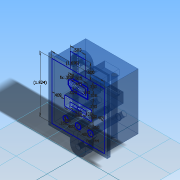
# Autodesk Inventor part: PanelMountNew
Saved by Autodesk Inventor 2014 SP2 (Build 180246200, 246)
## iProperties
Created: 2014-06-07
Part Number: PanelMountNew
Material: Generic
Document SubType Name: Modeling
Designer: dliu
Density: 1 g/cm^3
Appearance: Default
Author: dliu
Autodesk Inventor part; units mm, degrees
ref_plane "YZ Plane" through (0, 0, 0) normal (1, 0, 0) x (0, 1, 0)
ref_plane "XZ Plane" through (0, 0, 0) normal (0, 1, 0) x (-1, 0, 0)
sketch "Sketch1" plane through (0, 0, 0) normal (0, 0, 1) x (1, 0, 0)
  line L0 (7.6835, 18.4404) -> (7.6835, 10.414)
  line L1 (-7.6835, 15.9004) -> (-5.1435, 18.4404)
  line L2 (-7.6835, 12.954) -> (-5.1435, 10.414)
  line L3 (-7.6835, 12.954) -> (-7.6835, 15.9004)
  line L4 (-5.1435, 18.4404) -> (7.6835, 18.4404)
  line L5 (7.6835, 10.414) -> (-5.1435, 10.414)
  line L6 (-5.9055, 12.0142) -> (5.9055, 12.0142)
  line L7 (5.9055, 12.0142) -> (5.9055, 16.8402)
  line L8 (5.9055, 16.8402) -> (-5.9055, 16.8402)
  line L9 (-5.9055, 16.8402) -> (-5.9055, 12.0142)
  line L10 (-11.176, 4.064) -> (11.176, 4.064)
  line L11 (11.176, 4.064) -> (11.176, -4.064)
  line L12 (11.176, -4.064) -> (-11.176, -4.064)
  line L13 (-11.176, -4.064) -> (-11.176, 4.064)
  line L14 (-11.176, 4.064) -> (11.176, -4.064) construction
  line L15 (11.176, 4.064) -> (-11.176, -4.064) construction
  line L16 (-6.604, 1.27) -> (6.604, 1.27)
  line L17 (6.604, 1.27) -> (6.604, -1.27)
  line L18 (6.604, -1.27) -> (-6.604, -1.27)
  line L19 (-6.604, -1.27) -> (-6.604, 1.27)
  line L20 (-6.604, 1.27) -> (6.604, -1.27) construction
  line L21 (6.604, 1.27) -> (-6.604, -1.27) construction
  circle A0 centre (-10.16, -12.7952) radius 2.3813
  circle A1 centre (0, -12.7952) radius 2.3813
  circle A2 centre (10.16, -12.7952) radius 2.3813
  line L22 (-21.5583, 24.7904) -> (21.5583, 24.7904)
  line L23 (21.5583, 24.7904) -> (21.5583, -21.5265)
  line L24 (21.5583, -21.5265) -> (-21.5583, -21.5265)
  line L25 (-21.5583, -21.5265) -> (-21.5583, 24.7904)
  circle A3 centre (-10.16, -12.7952) radius 2.032
  circle A4 centre (0, -12.7952) radius 2.032
  circle A5 centre (10.16, -12.7952) radius 2.032
  line L26 (-7.6835, 14.4272) -> (7.6835, 14.4272) construction
  line L27 (5.9055, 12.0142) -> (-5.9055, 16.8402) construction
  line L28 (-5.3539, 9.906) -> (-8.1915, 12.7436)
  line L29 (-8.1915, 12.7436) -> (-8.1915, 16.1108)
  line L30 (-8.1915, 16.1108) -> (-5.3539, 18.9484)
  line L31 (-5.3539, 18.9484) -> (8.1915, 18.9484)
  line L32 (8.1915, 18.9484) -> (8.1915, 9.906)
  line L33 (8.1915, 9.906) -> (-5.3539, 9.906)
  point P0 (0, 0)
  point P1 (0, 0)
  point P2 (0, 0)
  point P3 (0, 14.4272)
  point P4 (0, 0)
  dimension "d1" = 8.0264
  dimension "d6" = 11.811
  dimension "d7" = 4.826
  dimension "d8" = 22.352
  dimension "d9" = 8.128
  dimension "d10" = 13.208
  dimension "d11" = 2.54
  dimension "d12" = 4.7625
  dimension "d13" = 10.16
  dimension "d14" = 10.16
  dimension "d15" = 6.35
  dimension "d18" = 8.7312
  dimension "d19" = 10.3823
  dimension "d20" = 10.3823
  dimension "d25" = 4.064
  dimension "d36" = 15.367
  dimension "d37" = 6.35
  dimension "d38" = 6.35
  dimension "d39" = 2.54
  dimension "d40" = 2.54
  dimension "d42" = 0.508
  dimension "d71" = 43.1167
  dimension "d72" = 46.3169
  constraints: 68 end point, 10 midpoint, 10 parallel, 8 perpendicular, 6 centre point, 5 coincident, 4 equal radius, 4 horizontal, 3 vertical alignment, 2 horizontal alignment, 5 other
  measures "d1" distance of L0.start L5.start
  measures "d6" distance of L9.start L7.end
  measures "d7" distance of L7.end L6.end
  measures "d8" distance of L12.start L13.start
  measures "d9" distance of L15.start L12.start
  measures "d10" distance of L18.start L19.start
  measures "d11" distance of L16.end L18.start
  measures "d12" diameter of A0
  measures "d13" distance of A1.centre A0.centre
  measures "d14" distance of A2.centre A1.centre
  measures "d15" distance edge to line of A1 L12
  measures "d18" distance from line of A2.centre L24
  measures "d19" distance between parallel lines of L13 L25
  measures "d20" distance between parallel lines of L23 L11
  measures "d25" diameter of A3
  measures "d36" distance between parallel lines of L0 L3
  measures "d37" distance between parallel lines of L10 L5
  measures "d38" distance between parallel lines of L4 L22
  measures "d39" horizontal distance of L3.end L1.end
  measures "d40" horizontal distance of L1.end L3.end
  measures "d42" distance between parallel lines of L33 L5
  measures "d71" distance of L22.start L22.end
  measures "d72" distance of L24.end L22.start
extrude "Base" add sketch "Sketch1" against normal blind 27.94 contours L0 L5 L2 L3 L1 L4 | L9 L8 L7 L6 | L10 L11 L12 L13 | L16 L17 L18 L19 | A0 | A1 | A2 | L22 L23 L24 L25 | A3 | A4 | A5 | L28 L29 L30 L31 L32 L33
sketch "Sketch3" plane through (0, 0, 0) normal (0, 0, 1) x (1, 0, 0)
  line L0 (-21.5583, 24.7904) -> (21.5583, 24.7904) projected
  line L1 (-21.5583, -21.5265) -> (-21.5583, 24.7904) projected
  line L2 (21.5583, -21.5265) -> (-21.5583, -21.5265) projected
  line L3 (21.5583, 24.7904) -> (21.5583, -21.5265) projected
  line L4 (24.0983, 27.3304) -> (-24.0983, 27.3304)
  line L5 (-24.0983, 27.3304) -> (-24.0983, -24.0665)
  line L6 (-24.0983, -24.0665) -> (24.0983, -24.0665)
  line L7 (24.0983, -24.0665) -> (24.0983, 27.3304)
  dimension "d54" = 2.54
  constraints: 8 end point, 3 other
  measures "d54" distance between parallel lines of L4 L0
extrude "Flange" add sketch "Sketch3" against normal blind 2.54
sketch "Sketch4" plane through (0, 0, 0) normal (0, 0, 1) x (1, 0, 0)
  line L0 (-21.5583, 24.7904) -> (21.5583, 24.7904) projected
  line L1 (-6.35, 37.4904) -> (6.35, 37.4904)
  line L2 (6.35, 37.4904) -> (6.35, 24.7904)
  line L3 (6.35, 24.7904) -> (-6.35, 24.7904)
  line L4 (-6.35, 24.7904) -> (-6.35, 37.4904)
  line L5 (0, 37.4904) -> (0, 24.7904) construction
  point P0 (0, 31.1404)
  dimension "d57" = 12.7
  dimension "d58" = 12.7
  constraints: 10 end point, 4 midpoint, 2 parallel, 1 horizontal, 1 perpendicular, 1 point on line
  measures "d57" distance of L2.end L3.end
  measures "d58" distance between parallel lines of L0 L1
extrude "Mounting Tab" add sketch "Sketch4" against normal blind 6.35
hole "Mounting Hole" at (0, 31.1404, 0) direction (0, 0, -1) diameter 3.81 end through all clearance for "Flat Head Machine Screw (82)" size "#6" standard "Ansi Unified Screw Threads"
fillet "Fillet1" radius 6.35 2 edges at (-6.35, 37.4904, -3.175) (6.35, 37.4904, -3.175)
ref_plane "Work Plane1" through (-21.5583, 1.6319, -27.94) normal (0, -1, 0) x (1, 0, 0)
mirror "Mirror3" about plane through (-21.5583, 1.6319, -27.94) normal (0, -1, 0) of "Mounting Tab", "Mounting Hole", "Fillet1"
fillet "Fillet2" radius 3.175 2 edges at (0, 24.7904, -6.35) (0, -21.5265, -6.35)
extrude "Bullet" cut sketch "Sketch1" against normal blind 23.114 contours A0 | A1 | A2 | A3 | A4 | A5
extrude "Bullet Wire" cut sketch "Sketch1" against normal through all contours A3 | A4 | A5
extrude "Balance" cut sketch "Sketch1" against normal blind 26.162 contours L10 L11 L12 L13 | L16 L17 L18 L19
extrude "Balance Wire" cut sketch "Sketch1" against normal through all contours L16 L17 L18 L19
extrude "XT60 Holder" cut sketch "Sketch1" against normal blind 18.3896 contours L0 L5 L2 L3 L1 L4 | L9 L8 L7 L6
extrude "XT60 Wire" cut sketch "Sketch1" against normal through all contours L9 L8 L7 L6
extrude "XT60 Shroud Space" cut sketch "Sketch1" against normal blind 10.6172 contours L0 L5 L2 L3 L1 L4 | L9 L8 L7 L6 | L28 L29 L30 L31 L32 L33
sketch "Sketch2" plane through (-21.5583, 24.7904, 0) normal (0, 1, 0) x (1, 0, 0)
  point P0 (21.5583, 0)
  point P1 (5.5563, 13.97)
  dimension "d45" = 13.97
  dimension "d46" = 16.002
  measures "d45" vertical distance of point (21.558, 0) point (5.556, 13.97)
  measures "d46" horizontal distance of point (21.558, 0) point (5.556, 13.97)
hole "Hole1" at (-16.002, 24.7904, -13.97) direction (0, -1, 0) diameter 3.81 end through all clearance for "Flat Head Machine Screw (82)" size "#6" standard "Ansi Unified Screw Threads"
mirror "Mirror1" about plane through (0, 0, 0) normal (1, 0, 0) of "Hole1"
equation "\"d15\" = d37"
equation "\"d18\" = d38 + 0.5 * d12"
equation "\"d20\" = d19"
equation "\"d40\" = d39"
body "Solid1"
